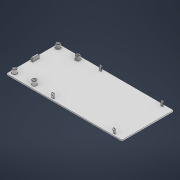
# Autodesk Inventor part: BOT
Saved by Autodesk Inventor 2022 (Build 260153000, 153)
## iProperties
Created: 2022-10-04
Part Number: BOT
Material: 常规
Document SubType Name: Modeling
Designer: 15628
Density: 1 g/cm^3
Appearance: 默认
Author: 15628
Autodesk Inventor part; units mm, degrees
ref_plane "YZ Plane" through (0, 0, 0) normal (1, 0, 0) x (0, 1, 0)
ref_plane "XZ Plane" through (0, 0, 0) normal (0, 1, 0) x (-1, 0, 0)
ref_plane "XY Plane" through (0, 0, 0) normal (0, 0, 1) x (1, 0, 0)
sketch "草图1" plane through (0, 0, 0) normal (0, 1, 0) x (-1, 0, 0)
  line L0 (0, 0) -> (145, 0)
  line L1 (145, 0) -> (145, -65)
  line L2 (145, -65) -> (0, -65)
  line L3 (0, -65) -> (0, 0)
  dimension "d0" = 145
  dimension "d1" = 65
  constraints: 8 end point, 2 parallel, 1 horizontal, 1 perpendicular
  measures "d0" distance of L1.end L2.end
  measures "d1" distance of L0.end L1.end
extrude "拉伸1" add sketch "草图1" along normal blind 2
sketch "草图2" plane through (0, 2, 0) normal (0, 1, 0) x (1, 0, 0)
  line L0 (-145, 0) -> (0, 0) projected
  line L1 (0, 0) -> (0, 2)
  line L2 (0, 0) -> (0, 65) projected
  line L3 (0, 2) -> (-12, 2)
  line L4 (-12, 2) -> (-12, 63)
  line L5 (-12, 2) -> (-89, 2)
  line L6 (-89, 2) -> (-89, 63)
  line L7 (-12, 2) -> (-12.9, 2)
  line L8 (-12.9, 2) -> (-12.9, 3)
  line L9 (-12.9, 3) -> (-11.1, 3)
  line L10 (-11.1, 3) -> (-11.1, 2)
  line L11 (-12, 63) -> (-12.9, 63)
  line L12 (-12.9, 63) -> (-12.9, 62)
  line L13 (-12.9, 62) -> (-11.1, 62)
  line L14 (-11.1, 62) -> (-11.1, 63)
  line L15 (-11.1, 63) -> (-12, 63)
  line L16 (-89, 63) -> (-88.1, 63)
  line L17 (-88.1, 63) -> (-88.1, 62)
  line L18 (-88.1, 62) -> (-89.9, 62)
  line L19 (-89.9, 62) -> (-89.9, 63)
  line L20 (-89.9, 63) -> (-88.1, 63)
  line L21 (-89, 2) -> (-89.9, 2)
  line L22 (-89.9, 2) -> (-89.9, 3)
  line L23 (-89.9, 3) -> (-88.1, 3)
  line L24 (-88.1, 3) -> (-88.1, 2)
  dimension "d4" = 2
  dimension "d5" = 12
  dimension "d6" = 61
  dimension "d7" = 77
  dimension "d8" = 0.9
  dimension "d9" = 1
  dimension "d10" = 1.8
  dimension "d11" = 1
  dimension "d12" = 0.9
  dimension "d13" = 1.8
  constraints: 46 end point, 14 perpendicular, 13 point on line, 2 parallel, 1 horizontal
  measures "d4" distance of L0.end L1.end
  measures "d5" distance of L1.end L3.end
  measures "d6" distance of L3.end L4.end
  measures "d7" distance of L3.end L5.end
  measures "d8" distance of L3.end L7.end
  measures "d9" distance of L7.end L8.end
  measures "d10" distance of L8.end L9.end
  measures "d11" distance of L11.end L12.end
  measures "d12" distance of L6.end L16.end
  measures "d13" distance of L17.end L18.end
extrude "拉伸2" add sketch "草图2" along normal blind 6
sketch "草图3" plane through (-89.9, 2, -3) normal (-1, 0, 0) x (0, 0, 1)
  line L0 (1, 0) -> (1, 6) projected
  line L1 (1, 6) -> (1, 4)
  line L2 (1, 4) -> (2, 4)
  line L3 (2, 4) -> (1, 6)
  line L4 (-60, 6) -> (-59, 6) projected
  line L5 (-60, 6) -> (-60, 4)
  line L6 (-60, 0) -> (-60, 6) projected
  line L7 (-60, 4) -> (-61, 4)
  line L8 (-61, 4) -> (-60, 6)
  point P0 (3, -2)
  dimension "d16" = 2
  dimension "d17" = 1
  dimension "d18" = 1
  constraints: 12 end point, 4 point on line, 1 perpendicular
  measures "d16" distance of L0.end L1.end
  measures "d17" distance of L1.end L2.end
  measures "d18" distance of L5.end L7.end
extrude "拉伸3" add sketch "草图3" against normal blind 1.8
sketch "草图4" plane through (-12.9, 2, -3) normal (-1, 0, 0) x (0, 0, 1)
  line L0 (1, 6) -> (2, 4) projected
  line L1 (2, 4) -> (1, 4) projected
  line L2 (1, 6) -> (2, 4)
  line L3 (2, 4) -> (1, 4)
  line L4 (1, 0) -> (1, 6) projected
  line L5 (1, 4) -> (1, 6)
  line L6 (-59, 6) -> (-60, 6) projected
  line L7 (-60, 6) -> (-60, 4)
  line L8 (-60, 0) -> (-60, 6) projected
  line L9 (-61, 4) -> (-60, 4) projected
  line L10 (-60, 6) -> (-61, 4) projected
  line L11 (-61, 4) -> (-60, 6)
  line L12 (-60, 0) -> (-60, 4) projected
  line L13 (-60, 6) -> (-60, 4)
  line L14 (-60, 4) -> (-61, 4)
  line L15 (1, 6) -> (0, 6) projected
  line L16 (1, 6) -> (1, 4)
  line L17 (1, 4) -> (2, 4)
  point P0 (3, -2)
  constraints: 18 end point, 3 perpendicular, 2 collinear, 1 horizontal, 1 point on line
extrude "拉伸4" add sketch "草图4" against normal blind 1.8
chamfer "倒角1" distance 0.5 angle 45 20 edges at (-72.5, 0, 0) (-145, 1, 0) (-145, 0, -32.5) (0, 1, 0) (-145, 1, -65) (-72.5, 0, -65) (0, 1, -65) (0, 0, -32.5) (-89, 2, -62) (-12, 2, -62) (-11.1, 2, -62.5) (-88.1, 2, -62.5) (-11.1, 2, -2.5) (-88.1, 2, -2.5) (-12.9, 2, -62.5) (-89.9, 2, -62.5) (-89.9, 2, -2.5) (-12.9, 2, -2.5) (-12, 2, -3) (-89, 2, -3)
sketch "草图5" plane through (0, 2, 0) normal (0, 1, 0) x (1, 0, 0)
  line L0 (-145, 64.5) -> (-145, 0.5) projected
  line L1 (-145, 64.5) -> (-143, 64.5)
  line L2 (-0.5, 64.5) -> (-144.5, 64.5) projected
  line L3 (-0.5, 65) -> (-144.5, 65) projected
  line L4 (-143, 65) -> (-115, 65)
  line L5 (-143, 65) -> (-143, 37)
  line L6 (-143, 37) -> (-143, 29)
  line L7 (-143, 37) -> (-141, 37)
  line L8 (-141, 37) -> (-141, 29)
  line L9 (-141, 29) -> (-143, 29)
  point P0 (0, 0)
  dimension "d26" = 2
  dimension "d27" = 28
  dimension "d28" = 28
  dimension "d29" = 8
  dimension "d30" = 2
  constraints: 14 end point, 4 point on line, 3 perpendicular, 1 horizontal
  measures "d26" distance of L0.start L1.end
  measures "d27" distance of L4.start L4.end
  measures "d28" distance of L4.start L5.end
  measures "d29" distance of L5.end L6.end
  measures "d30" distance of L5.end L7.end
extrude "拉伸5" add sketch "草图5" along normal blind 4
sketch "草图6" plane through (-143, 2, -29) normal (0, 0, 1) x (1, 0, 0)
  line L0 (0, 4) -> (2, 4) projected
  line L1 (0, 4) -> (0, 2)
  line L2 (0, 0) -> (0, 4) projected
  line L3 (0, 2) -> (-1, 2)
  line L4 (-1, 2) -> (0, 4)
  point P0 (143, -2)
  dimension "d33" = 2
  dimension "d34" = 1
  constraints: 6 end point, 1 midpoint, 1 perpendicular
  measures "d33" distance of L0.start L1.end
  measures "d34" distance of L1.end L3.end
extrude "拉伸6" add sketch "草图6" against normal blind 8
chamfer "倒角2" distance 0.5 angle 45 3 edges at (-141, 2, -33) (-142, 2, -29) (-142, 2, -37)
sketch "草图7" plane through (0, 2, 0) normal (0, 1, 0) x (1, 0, 0)
  line L0 (-144.5, 65) -> (-145, 64.5) projected
  line L1 (-145, 64.5) -> (-140.3, 64.5)
  line L2 (-0.5, 64.5) -> (-144.5, 64.5) projected
  line L3 (-140.3, 64.5) -> (-140.3, 65)
  line L4 (-0.5, 65) -> (-144.5, 65) projected
  line L5 (-140.3, 65) -> (-140.3, 60.3)
  line L6 (-140.3, 60.3) -> (-140.3, 5.6)
  line L7 (-140.3, 5.6) -> (-115.535, 5.6)
  line L8 (-115.535, 5.6) -> (-115.535, 60.3)
  line L9 (-115.535, 60.3) -> (-140.3, 60.3)
  circle A0 centre (-140.3, 60.3) radius 1.6
  circle A1 centre (-140.3, 60.3) radius 2.5
  circle A2 centre (-115.535, 60.3) radius 1.6
  circle A3 centre (-115.535, 60.3) radius 2.5
  circle A4 centre (-115.535, 5.6) radius 1.6
  circle A5 centre (-115.535, 5.6) radius 2.5
  circle A6 centre (-140.3, 5.6) radius 1.6
  circle A7 centre (-140.3, 5.6) radius 2.5
  point P0 (0, 0)
  dimension "d40" = 4.7
  dimension "d41" = 4.7
  dimension "d44" = 54.7
  dimension "d45" = 24.765
  dimension "d46" = 3.2
  dimension "d47" = 5
  dimension "d48" = 3.2
  dimension "d49" = 5
  dimension "d50" = 3.2
  dimension "d51" = 5
  dimension "d52" = 3.2
  dimension "d53" = 5
  constraints: 14 end point, 8 centre point, 8 coincident, 4 perpendicular, 3 point on line, 1 vertical
  measures "d40" distance of L0.end L1.end
  measures "d41" distance of L3.end L5.end
  measures "d44" distance of L5.end L6.end
  measures "d45" distance of L6.end L7.end
  measures "d46" diameter of A0
  measures "d47" diameter of A1
  measures "d48" diameter of A2
  measures "d49" diameter of A3
  measures "d50" diameter of A4
  measures "d51" diameter of A5
  measures "d52" diameter of A6
  measures "d53" diameter of A7
extrude "拉伸7" add sketch "草图7" along normal blind 5 contours A1 L9 A0 L5 | L5 A0 L6 A1 | A1 L6 A0 L9 | A3 L8 A2 L9 | L9 A2 L8 A3 | A7 L7 A6 L6 | L6 A6 L7 A7 | A5 L7 A4 L8 | L8 A4 L7 A5
chamfer "倒角3" distance 0.5 angle 45 13 edges at (-142.8, 2, -60.3) (-118.035, 2, -60.3) (-142.8, 2, -5.6) (-118.035, 2, -5.6) (-141.9, 7, -5.6) (-117.135, 7, -5.6) (-141.9, 7, -60.3) (-117.135, 7, -60.3) (-141, 6, -33) (-89, 8, -62) (-12, 8, -62) (-12, 8, -3) (-89, 8, -3)
